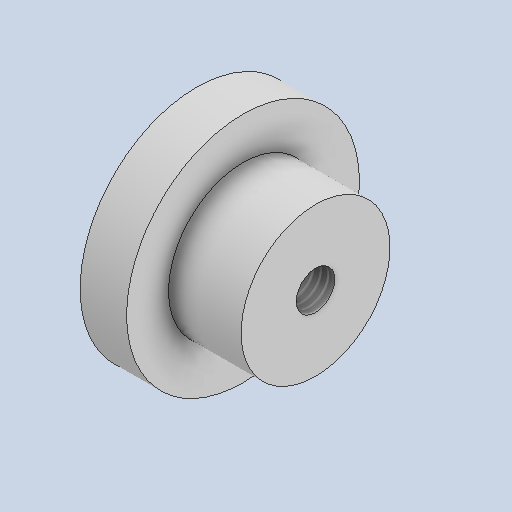
# Autodesk Inventor part: SpringCompensation_Outside_SupportPart
Saved by Autodesk Inventor 2022 (Build 260153000, 153)
## iProperties
Created: 2022-10-13
Part Number: SpringCompensation_Outside_SupportPart
Material: Generisch
Document SubType Name: Modeling
Designer: alexw
Density: 1 g/cm^3
Appearance: Vorgabe
Mass: 3.85085 g
Surface Area: 19.0591 cm^2
Volume: 3.85085 cm^3
Author: alexw
Autodesk Inventor part; units mm, degrees
ref_plane "YZ Plane" through (0, 0, 0) normal (1, 0, 0) x (0, 1, 0)
ref_plane "XZ Plane" through (0, 0, 0) normal (0, 1, 0) x (-1, 0, 0)
ref_plane "XY Plane" through (0, 0, 0) normal (0, 0, 1) x (1, 0, 0)
sketch "Skizze1" plane through (0, 0, 0) normal (0, 0, 1) x (1, 0, 0)
  line L0 (0, 0) -> (0, 12.5)
  line L1 (0, 12.5) -> (5, 12.5)
  line L2 (5, 12.5) -> (5, 8)
  line L3 (5, 8) -> (12.8, 8)
  line L4 (0, 0) -> (12.8, 0)
  line L5 (12.8, 8) -> (12.8, 0)
  dimension "d0" = 16
  dimension "d1" = 25
  dimension "d3" = 5
  dimension "d13" = 7.8
  constraints: 12 end point, 4 perpendicular, 1 horizontal, 1 vertical
  measures "d0" diameter of L3 L4
  measures "d1" diameter of L1 L4
  measures "d3" distance between parallel lines of L0 L2
  measures "d13" distance between parallel lines of L2 L5
revolve "Umdrehung1" add sketch "Skizze1" angle 360 about axis through (0, 0, 0) along (1, 0, 0)
sketch "Skizze2" plane through (0, 0, 0) normal (-1, 0, 0) x (0, 0, 1)
  point P0 (0, 0)
  point P1 (0, 0)
  constraints: 1 coincident
hole "Bohrung1" at (0, 0, 0) direction (1, 0, 0) diameter 4.134 end through all thread size "M5x0.8" class "6H" standard "ISO Metric profile"
feature "Verdickung1" [suppressed]
